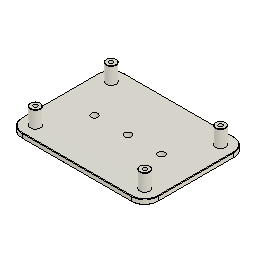
perf baord holder (Autodesk Fusion 360 design; units mm, degrees)
Autodesk Fusion 360 part; units mm, degrees
note: some values were not read from the file. Chosen so that the rebuilt part matches the saved one: which bodies a step acts on.
sketch "Sketch1" plane through (0, 0, 0) normal (0, 0, 1) x (1, 0, 0)
  line L0 (35, 25) -> (-35, 25)
  line L1 (-35, 25) -> (-35, -25)
  line L2 (-35, -25) -> (35, -25)
  line L3 (35, -25) -> (35, 25)
  line L4 (35, 25) -> (-35, -25) construction
  line L5 (-35, 25) -> (35, -25) construction
  circle A0 centre (-32.65, 22.65) radius 1.35
  line L6 (-34, 24) -> (-31.3, 24) construction
  line L7 (-31.3, 24) -> (-31.3, 21.3) construction
  line L8 (-31.3, 21.3) -> (-34, 21.3) construction
  line L9 (-34, 21.3) -> (-34, 24) construction
  line L10 (-34, 24) -> (-31.3, 21.3) construction
  line L11 (-31.3, 24) -> (-34, 21.3) construction
  line L12 (-35, 0) -> (35, 0) construction
  line L13 (0, 25) -> (0, -25) construction
  circle A1 centre (-32.65, -22.65) radius 1.35
  circle A2 centre (32.65, -22.65) radius 1.35
  circle A3 centre (32.65, 22.65) radius 1.35
  point P0 (-32.65, 22.65)
  dimension "d1" = 70
  dimension "d2" = 50
  dimension "d6" = 2.7
  dimension "d7" = 1
  dimension "d8" = 1
  constraint horizontal L0
  constraint perpendicular L0 L1
  constraint parallel L0 L2
  constraint parallel L1 L3
  constraint coincident L4 origin
  constraint coincident L5 origin
  constraint horizontal L6
  constraint perpendicular L6 L7
  constraint parallel L6 L8
  constraint parallel L7 L9
  constraint coincident L10 P0
  constraint coincident L11 P0
  constraint coincident P0 A0.centre
  constraint tangent A0 L6
  constraint tangent A0 L9
  constraint midpoint L1 L12.start
  constraint midpoint L3 L12.end
  constraint coincident L0 L13.start
  constraint midpoint L2 L13.end
  constraint symmetric A0 L12 A1
  constraint symmetric A0 L13 A3
  constraint symmetric L13 A1 A2
  constraint vertical L13
  measures "d1" distance of L1.end L2.end
  measures "d2" distance of L0.end L1.end
  measures "d6" diameter of A0
  measures "d7" distance of L1 L9
  measures "d8" distance of L0 L6
extrude "Extrude1" add sketch "Sketch1" along normal blind 1.5 makes body 1
sketch "Sketch2" plane through (0, 0, 0) normal (0, 0, 1) x (1, 0, 0)
  circle A0 centre (32.65, -22.65) radius 1.35
  circle A1 centre (-32.65, 22.65) radius 1.35
  circle A2 centre (-32.65, -22.65) radius 1.35
  circle A3 centre (32.65, 22.65) radius 1.35
  line L0 (35, -25) -> (35, 25)
  line L1 (35, 25) -> (-35, 25)
  line L2 (-35, 25) -> (-35, -25)
  line L3 (-35, -25) -> (35, -25)
  circle A4 centre (32.65, -22.65) radius 0.95
  circle A5 centre (32.65, 22.65) radius 0.95
  circle A6 centre (-32.65, 22.65) radius 0.95
  circle A7 centre (-32.65, -22.65) radius 0.95
  circle A8 centre (-32.65, -22.65) radius 3
  circle A9 centre (-32.65, 22.65) radius 3
  circle A10 centre (32.65, 22.65) radius 3
  circle A11 centre (32.65, -22.65) radius 3
  dimension "d11" = 1.9
  dimension "d12" = 1.9
  dimension "d13" = 1.9
  dimension "d14" = 1.9
  dimension "d15" = 6
  dimension "d16" = 6
  dimension "d17" = 6
  dimension "d18" = 6
  constraint concentric A0 A4
  constraint concentric A3 A5
  constraint concentric A1 A6
  constraint concentric A2 A7
  constraint concentric A7 A8
  constraint concentric A1 A9
  constraint concentric A5 A10
  constraint concentric A0 A11
  measures "d11" diameter of A4
  measures "d12" diameter of A5
  measures "d13" diameter of A6
  measures "d14" diameter of A7
  measures "d15" diameter of A8
  measures "d16" diameter of A9
  measures "d17" diameter of A10
  measures "d18" diameter of A11
extrude "Extrude1'" add sketch "Sketch2" against normal blind 10 separate body contours A0 | A1 | A2 | A3 | L0 L3 A11 | L0 A11 | L3 A11 | L0 L1 A10 | L0 A10 | L3 A8 | L2 L3 A8 | L1 A10 | L1 L2 A9 | L1 A9 | L2 A8 | L2 A9 picked at (32.6164, -24.6654) picked at (32.6164, 24.6654) picked at (-32.6836, -24.6654) picked at (-32.6836, 24.6654) makes body 2 at (35.6463, -22.7995, -6.6667) makes body 3 at (-29.6649, 22.9487, -3.3333) makes body 4 at (35.6351, 22.9487, -3.3333) makes body 5 at (-29.6649, -22.3513, -3.3333) in component "Component"
sketch "Sketch3" plane through (0, 0, -10) normal (0, 0, -1) x (1, 0, 0)
  circle A0 centre (32.65, -22.65) radius 0.95
  circle A1 centre (32.65, -22.65) radius 3 construction
  circle A2 centre (32.65, -22.65) radius 3
  circle A3 centre (-32.65, 22.65) radius 3 construction
  circle A4 centre (-32.65, -22.65) radius 3 construction
  circle A5 centre (32.65, 22.65) radius 3 construction
  line L0 (-32.65, 25.65) -> (32.65, 25.65)
  line L1 (35.65, 22.65) -> (35.65, -22.65)
  line L2 (32.65, -25.65) -> (-32.65, -25.65)
  line L3 (-35.65, 22.65) -> (-35.65, -22.65)
  arc A6 (35.65, 22.65) -> (32.65, 25.65) centre (32.65, 22.65) ccw
  arc A7 (32.65, -25.65) -> (35.65, -22.65) centre (32.65, -22.65) ccw
  arc A8 (-35.65, -22.65) -> (-32.65, -25.65) centre (-32.65, -22.65) ccw
  arc A9 (-32.65, 25.65) -> (-35.65, 22.65) centre (-32.65, 22.65) ccw
  arc A10 (40.65, 22.65) -> (32.65, 30.65) centre (32.65, 22.65) ccw
  line L4 (-32.65, 30.65) -> (32.65, 30.65)
  arc A11 (-32.65, 30.65) -> (-40.65, 22.65) centre (-32.65, 22.65) ccw
  line L5 (-40.65, 22.65) -> (-40.65, -22.65)
  arc A12 (-40.65, -22.65) -> (-32.65, -30.65) centre (-32.65, -22.65) ccw
  line L6 (32.65, -30.65) -> (-32.65, -30.65)
  arc A13 (32.65, -30.65) -> (40.65, -22.65) centre (32.65, -22.65) ccw
  line L7 (40.65, 22.65) -> (40.65, -22.65)
  dimension "d21" = -5
  constraint coincident A3 L0.start
  constraint coincident A5 L0.end
  constraint tangent A5 L0
  constraint horizontal L0
  constraint coincident A5 L1.start
  constraint coincident A2 L1.end
  constraint tangent A2 L1
  constraint perpendicular L0 L1
  constraint coincident A1 L2.start
  constraint coincident A4 L2.end
  constraint tangent A4 L2
  constraint tangent A1 L2
  constraint coincident A3 L3.start
  constraint coincident A4 L3.end
  constraint tangent A4 L3
  constraint perpendicular L0 L3
extrude "Extrude2" add sketch "Sketch3" along normal blind 3 contours A0 | A2 A7 | A2 L0 L1 L2 L3 A6 A8 A9 | A10 L4 A11 L5 A12 L6 A13 L7 bodies 2 5 4 3 in component "Component"
copy_body "Body->Comp1" bodies 1 removing the originals makes body 6 in component "Component'"
fillet "Fillet1" radius 0.3 16 edges at (-38.3069, 28.3069, -10) (-40.65, 0, -10) (-38.3069, -28.3069, -10) (0, -30.65, -10) (38.3069, -28.3069, -10) (40.65, 0, -10) (38.3069, 28.3069, -10) (0, 30.65, -10) (40.65, 0, -13) (38.3069, -28.3069, -13) (0, -30.65, -13) (-38.3069, -28.3069, -13) (-40.65, 0, -13) (-38.3069, 28.3069, -13) (0, 30.65, -13) (38.3069, 28.3069, -13) on bodies 2 in component "Component"
chamfer "Chamfer1" distance 0.2 distance2 2 4 edges at (31.7643, -22.3065, 0) (-33.5357, -22.3065, 0) (31.7643, 22.9935, 0) (-33.5357, 22.9935, 0) measured on face at (34.9555, -22.501, 0) measured on face at (-30.348, -22.4538, 0) measured on face at (34.9555, 22.799, 0) measured on face at (-30.3445, 22.799, 0) on bodies 2 in component "Component"
sketch "Sketch4" plane through (0, 0, -13) normal (0, 0, -1) x (1, 0, 0)
  line L0 (40.35, -22.65) -> (40.35, 22.65)
  arc A0 (40.35, 22.65) -> (32.65, 30.35) centre (32.65, 22.65) ccw
  line L1 (32.65, 30.35) -> (-32.65, 30.35)
  arc A1 (-32.65, 30.35) -> (-40.35, 22.65) centre (-32.65, 22.65) ccw
  line L2 (-40.35, 22.65) -> (-40.35, -22.65)
  arc A2 (-40.35, -22.65) -> (-32.65, -30.35) centre (-32.65, -22.65) ccw
  line L3 (-32.65, -30.35) -> (32.65, -30.35)
  arc A3 (32.65, -30.35) -> (40.35, -22.65) centre (32.65, -22.65) ccw
  circle A4 centre (20, 0) radius 2
  circle A5 centre (0, 0) radius 2
  circle A6 centre (-20, 0) radius 2
  point P0 (-20, 0)
  point P1 (20, 0)
  point P2 (40, 0)
  dimension "d30" = 20
  dimension "d31" = 0
  dimension "d32" = 4
  dimension "d33" = 4
  dimension "d34" = 4
  constraint coincident A5.centre origin
  constraint coincident P1 A4.centre
  constraint coincident P0 A6.centre
  measures "d32" diameter of A4
  measures "d33" diameter of A5
  measures "d34" diameter of A6
extrude "Extrude3" cut sketch "Sketch4" against normal blind 10 contours A4 | A5 | A6 bodies 2 in component "Component"
fillet "Fillet2" radius 0.2 4 edges at (-35.447, 21.5652, 0) (-35.447, -23.7348, 0) (29.853, -23.7348, 0) (29.853, 21.5652, 0) on bodies 2 in component "Component"
component "Component" placed x (1, 0, 0) y (0, 1, 0) z (0, 0, 1) at (0, 0, 0)
component "Component'" placed x (1, 0, 0) y (0, 1, 0) z (0, 0, 1) at (0, 0, 0)
